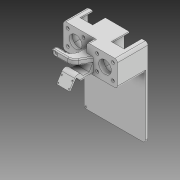
# Autodesk Inventor part: Base
Saved by Autodesk Inventor 2020 (Build 240168000, 168)
## iProperties
Created: 2020-07-24
Part Number: Base
Material: Generic
Document SubType Name: Modeling
Designer: DDeGo
Density: 1 g/cm^3
Appearance: Default
Author: DDeGo
Autodesk Inventor part; units mm, degrees
ref_plane "YZ Plane" through (0, 0, 0) normal (1, 0, 0) x (0, 1, 0)
ref_plane "XZ Plane" through (0, 0, 0) normal (0, 1, 0) x (-1, 0, 0)
ref_plane "XY Plane" through (0, 0, 0) normal (0, 0, 1) x (1, 0, 0)
sketch "Sketch1" plane through (0, 0, 0) normal (0, 0, 1) x (1, 0, 0)
  line L0 (-60.5, -85) -> (60.5, -85)
  line L1 (60.5, -85) -> (60.5, 85)
  line L2 (60.5, 85) -> (-60.5, 85)
  line L3 (-60.5, 85) -> (-60.5, -85)
  line L4 (-60.5, -85) -> (60.5, 85) construction
  line L5 (60.5, -85) -> (-60.5, 85) construction
  line L6 (-60.5, 35) -> (60.5, 35) construction
  line L7 (-57.5, 82) -> (-13.5, 82) construction
  line L8 (-13.5, 82) -> (-13.5, 38) construction
  line L9 (-13.5, 38) -> (-57.5, 38) construction
  line L10 (-57.5, 38) -> (-57.5, 82) construction
  line L11 (13.5, 82) -> (57.5, 82) construction
  line L12 (57.5, 82) -> (57.5, 38) construction
  line L13 (57.5, 38) -> (13.5, 38) construction
  line L14 (13.5, 38) -> (13.5, 82) construction
  point P0 (0, 0)
  dimension "d1" = 121
  dimension "d3" = 120
  dimension "d35" = 44
  dimension "d36" = 44
  dimension "d37" = 3
  dimension "d38" = 3
  dimension "d40" = 3
  dimension "d41" = 3
  dimension "d42" = 27
  constraints: 30 end point, 6 parallel, 4 perpendicular, 3 collinear, 3 horizontal, 2 midpoint, 2 point on line
  measures "d1" distance of L0.start L0.end
  measures "d3" distance between parallel lines of L0 L6
  measures "d35" distance between parallel lines of L8 L10
  measures "d36" distance between parallel lines of L7 L9
  measures "d37" distance between parallel lines of L6 L9
  measures "d38" distance between parallel lines of L2 L7
  measures "d40" distance between parallel lines of L3 L10
  measures "d41" distance between parallel lines of L1 L12
  measures "d42" distance between parallel lines of L8 L14
extrude "Extrusion1" add sketch "Sketch1" along normal blind 5
sketch "Sketch2" plane through (0, 0, 5) normal (0, 0, 1) x (1, 0, 0)
  line L0 (60.5, 85) -> (-60.5, 85) projected
  line L1 (60.5, -85) -> (60.5, 85) projected
  line L2 (-60.5, 85) -> (60.5, 85)
  line L3 (60.5, 85) -> (60.5, 35)
  line L4 (60.5, 35) -> (-60.5, 35)
  line L5 (-60.5, 35) -> (-60.5, 85)
  line L6 (-60.5, 35) -> (60.5, 35) construction
  point P0 (0, 0)
  constraints: 8 end point, 2 parallel, 2 point on line, 1 horizontal, 1 perpendicular
extrude "Extrusion2" add sketch "Sketch2" along normal blind 55
sketch "Sketch3" plane through (0, 0, 0) normal (0, 0, -1) x (-1, 0, 0)
  line L0 (-60.5, -85) -> (-60.5, 85) projected
  line L1 (-60.5, 60.5) -> (60.5, 60.5) construction
  line L2 (60.5, 85) -> (60.5, -85) projected
  line L3 (-14, 38.5) -> (-58, 38.5)
  line L4 (-58, 38.5) -> (-58, 82.5)
  line L5 (-58, 82.5) -> (-14, 82.5)
  line L6 (-14, 82.5) -> (-14, 38.5)
  line L7 (-14, 38.5) -> (-58, 82.5) construction
  line L8 (-58, 38.5) -> (-14, 82.5) construction
  line L9 (58, 38.5) -> (14, 38.5)
  line L10 (14, 38.5) -> (14, 82.5)
  line L11 (14, 82.5) -> (58, 82.5)
  line L12 (58, 82.5) -> (58, 38.5)
  line L13 (58, 38.5) -> (14, 82.5) construction
  line L14 (14, 38.5) -> (58, 82.5) construction
  line L15 (-60.5, 85) -> (60.5, 85) projected
  line L16 (-58, 38.5) -> (-60.5, 38.5) construction
  line L17 (58, 38.5) -> (60.5, 38.5) construction
  line L18 (60.5, 85) -> (60.5, 35) projected
  point P0 (0, 0)
  point P1 (-36, 60.5)
  point P2 (36, 60.5)
  dimension "d8" = 44
  dimension "d9" = 44
  dimension "d10" = 44
  dimension "d11" = 24.5
  dimension "d12" = 24.5
  dimension "d39" = 24.5
  dimension "d69" = 72
  constraints: 30 end point, 8 point on line, 4 midpoint, 4 parallel, 4 perpendicular, 2 horizontal, 1 collinear
  measures "d8" distance of L9.end L10.end
  measures "d9" distance of L10.end L11.end
  measures "d10" distance of L4.end L5.end
  measures "d11" distance from line of L0 point (-36, 60.5)
  measures "d12" distance from line of L2 point (36, 60.5)
  measures "d39" distance between parallel lines of L1 L15
  measures "d69" distance of point (-36, 60.5) point (36, 60.5)
extrude "Extrusion3" cut sketch "Sketch3" against normal blind 40
sketch "Sketch4" plane through (0, 0, 40) normal (0, 0, -1) x (-1, 0, 0)
  line L0 (-58, 38.5) -> (-58, 82.5) projected
  line L1 (-58, 82.5) -> (-14, 82.5) projected
  line L2 (-58, 38.5) -> (-14, 82.5) construction
  line L3 (14, 82.5) -> (58, 82.5) projected
  line L4 (58, 82.5) -> (58, 38.5) projected
  line L5 (14, 82.5) -> (58, 38.5) construction
  line L6 (-20.5, 76) -> (-51.5, 76) construction
  line L7 (-51.5, 76) -> (-51.5, 45) construction
  line L8 (-51.5, 45) -> (-20.5, 45) construction
  line L9 (-20.5, 45) -> (-20.5, 76) construction
  line L10 (-20.5, 76) -> (-51.5, 45) construction
  line L11 (-51.5, 76) -> (-20.5, 45) construction
  line L12 (51.5, 45) -> (20.5, 45) construction
  line L13 (20.5, 45) -> (20.5, 76) construction
  line L14 (20.5, 76) -> (51.5, 76) construction
  line L15 (51.5, 76) -> (51.5, 45) construction
  line L16 (51.5, 45) -> (20.5, 76) construction
  line L17 (20.5, 45) -> (51.5, 76) construction
  circle A0 centre (-51.5, 45) radius 1.75
  circle A1 centre (-51.5, 76) radius 1.75
  circle A2 centre (-20.5, 76) radius 1.75
  circle A3 centre (-20.5, 45) radius 1.75
  circle A4 centre (20.5, 76) radius 1.75
  circle A5 centre (20.5, 45) radius 1.75
  circle A6 centre (51.5, 76) radius 1.75
  circle A7 centre (51.5, 45) radius 1.75
  circle A8 centre (-36, 60.5) radius 12.5
  circle A9 centre (36, 60.5) radius 12.5
  point P0 (0, 0)
  dimension "d16" = 31
  dimension "d17" = 3.5
  dimension "d18" = 25
  dimension "d68" = 72
  constraints: 28 end point, 10 centre point, 10 coincident, 8 equal radius, 6 midpoint, 5 parallel, 2 horizontal, 2 perpendicular, 2 point on line
  measures "d16" distance of L12.end L13.end
  measures "d17" diameter of A0
  measures "d18" diameter of A9
  measures "d68" distance of A8.centre point (36, 60.5)
extrude "Extrusion4" cut sketch "Sketch4" against normal through all
sketch "Sketch5" plane through (0, 0, 0) normal (0, 0, -1) x (-1, 0, 0)
  line L0 (-58, 82.5) -> (-14, 82.5) construction
  line L1 (-36, 82.5) -> (-36, 85) construction
  line L2 (-60.5, 85) -> (60.5, 85) construction
  line L3 (14, 82.5) -> (58, 82.5) construction
  line L4 (36, 82.5) -> (36, 85) construction
  line L5 (-48.5, 85) -> (-23.5, 85)
  line L6 (-23.5, 85) -> (-23.5, 82.5)
  line L7 (-23.5, 82.5) -> (-48.5, 82.5)
  line L8 (-48.5, 82.5) -> (-48.5, 85)
  line L9 (-48.5, 85) -> (-23.5, 82.5) construction
  line L10 (-23.5, 85) -> (-48.5, 82.5) construction
  line L11 (48.5, 85) -> (23.5, 85)
  line L12 (23.5, 85) -> (23.5, 82.5)
  line L13 (23.5, 82.5) -> (48.5, 82.5)
  line L14 (48.5, 82.5) -> (48.5, 85)
  line L15 (48.5, 85) -> (23.5, 82.5) construction
  line L16 (23.5, 85) -> (48.5, 82.5) construction
  point P0 (0, 0)
  point P1 (-36, 83.75)
  point P2 (36, 83.75)
  dimension "d21" = 25
  constraints: 28 end point, 8 midpoint, 4 parallel, 4 point on line, 2 horizontal, 2 perpendicular, 2 vertical, 1 collinear
  measures "d21" distance between parallel lines of L6 L8
extrude "Extrusion5" cut sketch "Sketch5" against normal blind 25
sketch "Sketch6" plane through (0, 0, 60) normal (0, 0, 1) x (1, 0, 0)
  line L0 (-60.5, 85) -> (-60.5, 35) projected
  line L1 (-60.5, 35) -> (60.5, 35) projected
  line L2 (-60.5, 85) -> (0, 85)
  line L3 (0, 85) -> (0, 35)
  line L4 (0, 35) -> (-60.5, 35)
  line L5 (-60.5, 35) -> (-60.5, 85)
  point P0 (0, 0)
  constraints: 8 end point, 2 parallel, 1 horizontal, 1 midpoint, 1 perpendicular
extrude "Extrusion6" cut sketch "Sketch6" against normal blind 14
sketch "Sketch7" plane through (0, 0, 40) normal (0, 0, -1) x (-1, 0, 0)
  circle A0 centre (-51.5, 45) radius 1.75 projected
  circle A1 centre (-20.5, 45) radius 1.75 projected
  circle A2 centre (-36, 60.5) radius 12.5 projected
  circle A3 centre (-51.5, 76) radius 1.75 projected
  circle A4 centre (-20.5, 76) radius 1.75 projected
  line L0 (-14, 82.5) -> (-14, 38.5) projected
  line L1 (-58, 82.5) -> (-14, 82.5) projected
  line L2 (-58, 38.5) -> (-58, 82.5) projected
  line L3 (-14, 38.5) -> (-58, 38.5) projected
  point P0 (0, 0)
extrude "Extrusion7" cut sketch "Sketch7" against normal blind 10
sketch "Sketch8" plane through (0, 0, 46) normal (0, 0, 1) x (1, 0, 0)
  circle A0 centre (-51.5, 45) radius 1.75 projected
  circle A1 centre (-20.5, 45) radius 1.75 projected
  circle A2 centre (-20.5, 76) radius 1.75 projected
  circle A3 centre (-51.5, 76) radius 1.75 projected
  circle A4 centre (-51.5, 45) radius 3
  circle A5 centre (-51.5, 76) radius 3
  circle A6 centre (-20.5, 76) radius 3
  circle A7 centre (-20.5, 45) radius 3
  point P0 (0, 0)
  dimension "d28" = 6
  constraints: 4 centre point, 3 equal radius
  measures "d28" diameter of A4
extrude "Extrusion8" cut sketch "Sketch8" against normal blind 2.5 contours A0 | A1 | A2 | A3 | A4 | A5 | A6 | A7
sketch "Sketch9" plane through (0, 0, 60) normal (0, 0, 1) x (1, 0, 0)
  circle A0 centre (20.5, 45) radius 1.75 projected
  circle A1 centre (20.5, 76) radius 1.75 projected
  circle A2 centre (51.5, 76) radius 1.75 projected
  circle A3 centre (51.5, 45) radius 1.75 projected
  circle A4 centre (20.5, 45) radius 3
  circle A5 centre (20.5, 76) radius 3
  circle A6 centre (51.5, 76) radius 3
  circle A7 centre (51.5, 45) radius 3
  point P0 (0, 0)
  dimension "d31" = 6
  constraints: 4 centre point, 3 equal radius
  measures "d31" diameter of A4
extrude "Extrusion9" cut sketch "Sketch9" against normal blind 2.5 contours A0 | A1 | A2 | A3 | A4 | A5 | A6 | A7
sketch "Sketch10" plane through (0, 0, 46) normal (0, 0, 1) x (1, 0, 0)
  line L0 (0, 35) -> (-60.5, 35) projected
  line L1 (0, 35) -> (-12.5, 35)
  line L2 (-12.5, 35) -> (-12.5, 57)
  line L3 (-12.5, 57) -> (0, 57)
  line L4 (0, 57) -> (0, 35)
  circle A0 centre (-20.5, 45) radius 1.75 projected
  point P0 (0, 0)
  point P1 (-58, 35)
  dimension "d44" = 22
  dimension "d53" = 12.5
  constraints: 8 end point, 2 parallel, 1 horizontal, 1 perpendicular
  measures "d44" distance between parallel lines of L0 L3
  measures "d53" distance of L2.end L3.end
extrude "Extrusion10" add sketch "Sketch10" along normal up to surface (14 mm away) contours L0 L2 L3 L4
sketch "Sketch11" plane through (-12.5, 35, 46) normal (-1, 0, 0) x (0, 0, 1)
  line L0 (46, 10.8553) -> (57.264, -6.8683) construction
  line L1 (51.632, 1.9935) -> (-41, -56.8776) construction
  line L2 (0, 22) -> (14, 22) projected
  line L3 (0, 0) -> (0, 50) projected
  line L4 (-41, 0) -> (-41, -120) projected
  line L5 (48.3697, 10.8553) -> (58.9519, -5.7955)
  line L6 (58.9519, -5.7955) -> (57.264, -6.8683) construction
  line L7 (49.1, 0.3844) -> (-41, -18.2539) construction
  line L8 (-41, -120) -> (-41, 0) projected
  line L9 (49.1, 0.3844) -> (-41, -120) construction
  line L10 (58.9519, -5.7955) -> (61.4838, -4.1864)
  line L11 (61.4838, -4.1864) -> (50.7292, 12.7358)
  line L12 (14, 0) -> (14, 22) projected
  line L13 (14, 0) -> (14, 22)
  line L14 (46, 10.8553) -> (48.3697, 10.8553)
  line L15 (37.849, 13.5871) -> (34, 9)
  line L16 (34, 9) -> (22, 9)
  line L17 (0, 22) -> (14, 22) projected
  line L18 (22, 9) -> (14, 22)
  line L19 (46, 10.8553) -> (36.8914, 0)
  line L20 (36.8914, 0) -> (14, 0)
  arc A0 (50.7292, 12.7358) -> (37.849, 13.5871) centre (43.9774, 8.4448) ccw
  point P0 (-46, -35)
  dimension "d47" = 21
  dimension "d70" = 20.75
  dimension "d71" = 20.75
  dimension "d72" = 5
  dimension "d73" = 3
  dimension "d77" = 2
  dimension "d78" = 9
  dimension "d79" = 130
  dimension "d80" = 20
  dimension "d81" = 8
  dimension "d82" = 8
  dimension "d83" = 8
  dimension "d84" = 32
  constraints: 30 end point, 3 horizontal, 3 parallel, 3 perpendicular, 3 point on line, 2 point on circle, 2 tangent, 1 centre point, 1 midpoint, 1 vertical
  measures "d47" distance of L0.start L0.end
  measures "d70" angle of L7 L1
  measures "d71" angle of L9 L1
  measures "d72" distance from line of L5 L7.start
  measures "d73" distance between parallel lines of L5 L11
  measures "d77" distance between parallel lines of L0 L5
  measures "d78" distance from line of L12.start L16
  measures "d79" angle of L16 L15
  measures "d80" distance from line of L12 L15.end
  measures "d81" radius of A0
  measures "d82" distance from line of L12 L16.end
  measures "d83" distance between parallel lines of L19 L15
  measures "d84" distance from line of L12 L0.start
extrude "Extrusion11" add sketch "Sketch11" against normal blind 25
sketch "Sketch13" plane through (-12.5, 60.0552, 85.3452) normal (0, -0.536379, -0.8439773) x (1, 0, 0)
  line L0 (2.25, 21.3039) -> (22.75, 21.3039) construction
  line L1 (22.75, 21.3039) -> (22.75, 33.8039) construction
  line L2 (22.75, 33.8039) -> (2.25, 33.8039) construction
  line L3 (2.25, 33.8039) -> (2.25, 21.3039) construction
  line L4 (2.25, 21.3039) -> (22.75, 33.8039) construction
  line L5 (22.75, 21.3039) -> (2.25, 33.8039) construction
  circle A0 centre (2.25, 33.8039) radius 1.2
  circle A1 centre (2.25, 21.3039) radius 1.2
  circle A2 centre (22.75, 21.3039) radius 1.2
  circle A3 centre (22.75, 33.8039) radius 1.2
  line L6 (12.5, 27.5539) -> (12.5, 36.5539) construction
  line L7 (0, 36.5539) -> (25, 36.5539) projected
  point P0 (12.5, 4.9078)
  dimension "d59" = 2.4
  dimension "d60" = 12.5
  dimension "d61" = 20.5
  dimension "d85" = 9
  constraints: 14 end point, 4 centre point, 4 coincident, 3 equal radius, 2 midpoint, 2 parallel, 1 horizontal, 1 perpendicular, 1 vertical
  measures "d59" diameter of A1
  measures "d60" distance of L2.end L0.start
  measures "d61" distance of L0.start L0.end
  measures "d85" distance of L6.start L6.end
extrude "Extrusion13" cut sketch "Sketch13" against normal through all
sketch "Sketch15" plane through (12.5, 45.8553, 94.3697) normal (0, -0.536379, -0.8439773) x (-1, 0, 0)
  circle A0 centre (22.75, -16.9789) radius 1.2 projected
  line L0 (22.75, -16.9789) -> (2.25, -16.9789)
  line L1 (2.25, -16.9789) -> (2.25, 0)
  line L2 (2.25, 0) -> (22.75, 0)
  line L3 (22.75, 0) -> (22.75, -16.9789)
  circle A1 centre (2.25, -4.4789) radius 1.2 projected
  line L4 (25, 0) -> (0, 0) projected
  point P0 (12.5, 11.9171)
  point P1 (2.25, -3.2789)
  point P2 (2.25, -5.6789)
  point P3 (21.55, -16.9789)
  point P4 (22.75, -15.7789)
  constraints: 8 end point, 2 parallel, 1 collinear, 1 horizontal, 1 perpendicular, 1 point on line
extrude "Extrusion15" cut sketch "Sketch15" against normal blind 1.5 contours A0 L0 L1 A1 L2 L3
chamfer "Chamfer1" distance 0.75 angle 45 2 edges at (0, 31.5254, 103.4769) (0, 32.3311, 104.7445)
sketch "Sketch17" plane through (0, 0, 25) normal (0, 0, -1) x (-1, 0, 0)
  line L0 (-23.5, 82.5) -> (-48.5, 82.5) projected
  line L1 (-23.5, 85) -> (-23.5, 82.5) projected
  line L2 (-48.5, 85) -> (-23.5, 85) projected
  line L3 (-48.5, 82.5) -> (-48.5, 85) projected
  point P0 (0, 0)
extrude "Extrusion16" cut sketch "Sketch17" against normal blind 10
sketch "Sketch18" plane through (0, 0, 5) normal (0, 0, 1) x (1, 0, 0)
  circle A0 centre (-56.5, -81) radius 4 construction
  circle A1 centre (-56.5, -81) radius 1
  line L0 (-60.5, 35) -> (-60.5, -85) projected
  line L1 (-60.5, -85) -> (60.5, -85) projected
  point P0 (0, 0)
  point P1 (-60.5, 27.6863)
  dimension "d95" = 8
  dimension "d96" = 2
  constraints: 2 centre point, 2 tangent, 1 coincident
  measures "d95" diameter of A0
  measures "d96" diameter of A1
extrude "Extrusion17" cut sketch "Sketch18" against normal blind 3
chamfer "Chamfer2" distance 0.5 angle 45 1 edges at (-57.5, -81, 5)
ref_plane "Work Plane1" through (-58, 60.5, 0) normal (0, 1, 0) x (1, 0, 0)
sketch "Sketch19" plane through (-58, 60.5, 0) normal (0, 1, 0) x (1, 0, 0)
  line L0 (9.5, -46) -> (34.5, -46) projected
  line L1 (22, -46) -> (22, -77) construction
  line L2 (22, -77) -> (15, -77)
  line L3 (15, -77) -> (15, -86)
  line L4 (15, -86) -> (46.8286, -86)
  line L5 (70.5, -60) -> (70.5, -68) projected
  line L6 (59.819, -78.5) -> (70.5, -60)
  line L7 (58, -46) -> (58, -60) projected
  line L8 (70.5, -60) -> (58, -60)
  line L9 (58, -60) -> (58, -46)
  line L10 (58, -46) -> (45.5, -46)
  line L11 (45.5, -46) -> (45.5, -66.5981)
  line L12 (45.5, -46) -> (45.5, -82.8914) construction
  line L13 (34, -77) -> (22, -77)
  line L14 (34, -77) -> (40.5, -75.2583)
  line L15 (40.5, -75.2583) -> (45.5, -66.5981)
  arc A0 (46.8286, -86) -> (59.819, -78.5) centre (46.8286, -71) ccw
  point P0 (58, 0)
  point P1 (55.4889, -86)
  dimension "d103" = 31
  dimension "d105" = 9
  dimension "d106" = 150
  dimension "d107" = 15
  dimension "d108" = 5
  dimension "d121" = 15
  dimension "d122" = 7
  dimension "d123" = 12
  constraints: 24 end point, 4 perpendicular, 4 point on line, 3 collinear, 2 parallel, 2 point on circle, 2 tangent, 1 centre point, 1 midpoint, 1 vertical
  measures "d103" distance between parallel lines of L0 L2
  measures "d105" distance between parallel lines of L13 L4
  measures "d106" angle of L11 L15
  measures "d107" angle of L13 L14
  measures "d108" distance from line of L12 L14.end
  measures "d121" radius of A0
  measures "d122" distance of L1.end L2.end
  measures "d123" distance of L13.start L1.end
extrude "Extrusion18" add sketch "Sketch19" along normal mid plane 11
sketch "Sketch20" plane through (-24, 66, 77) normal (0, 0, -1) x (-1, 0, 0)
  circle A0 centre (12, -5.5) radius 2.65
  point P0 (-24, -66)
  dimension "d111" = 5.3
  constraints: 1 centre point, 1 coincident
  measures "d111" diameter of A0
extrude "Extrusion19" cut sketch "Sketch20" against normal through all
sketch "Sketch21" plane through (-24, 66, 77) normal (0, 0, -1) x (-1, 0, 0)
  circle A0 centre (12, -5.5) radius 2.65 projected
  line L0 (16.6765, -5.5) -> (14.3383, -9.55)
  line L1 (14.3383, -9.55) -> (9.6617, -9.55)
  line L2 (9.6617, -9.55) -> (7.3235, -5.5)
  line L3 (7.3235, -5.5) -> (9.6617, -1.45)
  line L4 (9.6617, -1.45) -> (14.3383, -1.45)
  line L5 (14.3383, -1.45) -> (16.6765, -5.5)
  point P0 (-24, -66)
  dimension "d114" = 8.1
  constraints: 12 end point, 1 coincident, 1 horizontal, 13 other
  measures "d114" distance between parallel lines of L4 L1
extrude "Extrusion20" [suppressed]
sketch "Sketch22" plane through (-2.5111, 55, 86) normal (0, 0, 1) x (1, 0, 0)
  circle A0 centre (-33.4889, 5.5) radius 2.65 projected
  circle A1 centre (-33.4889, 5.5) radius 4.5
  point P0 (2.5111, -55)
  dimension "d118" = 9
  constraints: 1 centre point, 1 coincident
  measures "d118" diameter of A1
extrude "Extrusion21" cut sketch "Sketch22" against normal blind 3.5
fillet "Fillet3" radius 3 14 edges at (-43, 66, 81.5) (-43, 55, 81.5) (-24, 60.5, 77) (-17.5, 60.5, 75.2583) (-12.5, 60.5, 66.5981) (-12.5, 66, 56.299) (-15, 66, 70.9282) (-20.75, 66, 76.1292) (-33.5, 66, 77) (-43, 60.5, 77) (-33.5, 55, 77) (-20.75, 55, 76.1292) (-15, 55, 70.9282) (-12.5, 55, 63.9144)
fillet "Fillet4" radius 5 9 edges at (-60.5, 85, 23) (-60.5, 35, 25.5) (60.5, 85, 30) (60.5, 35, 32.5) (-12.5, 35, 64.4457) (12.5, 35, 71.4457) (0, 85, 53) (-60.5, -85, 2.5) (60.5, -85, 2.5)
fillet "Fillet4" radius 2 9 edges at (7.1595, 66, 69.25) (-25.5857, 66, 86) (-42.1213, 65.1213, 86) (-43, 60.5, 86) (-42.1213, 55.8787, 86) (-25.5857, 55, 86) (-3.6714, 55, 83.9904) (6.8042, 55, 69.8654) (-3.6714, 66, 83.9904)
body "Solid1"
